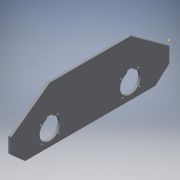
# Autodesk Inventor part: боковина
Saved by Autodesk Inventor 2019 (Build 230136000, 136)
## iProperties
Created: 2022-02-24
Part Number: боковина
Material: Типовые
Document SubType Name: Modeling
Designer: korsh
Density: 1 g/cm^3
Appearance: По умолчанию
Author: korsh
Autodesk Inventor part; units mm, degrees
ref_plane "YZ Plane" through (0, 0, 0) normal (1, 0, 0) x (0, 1, 0)
ref_plane "XZ Plane" through (0, 0, 0) normal (0, 1, 0) x (-1, 0, 0)
ref_plane "XY Plane" through (0, 0, 0) normal (0, 0, 1) x (1, 0, 0)
sketch "Эскиз1" plane through (0, 0, 0) normal (1, 0, 0) x (0, 1, 0)
  circle A0 centre (-34.2904, 95.1504) radius 32.5 projected
  circle A1 centre (-34.2904, 281.4981) radius 32.5 projected
  circle A2 centre (-13.0063, 263.3051) radius 2 projected
  circle A3 centre (-16.0973, 302.7822) radius 2 projected
  circle A4 centre (-55.5744, 299.6912) radius 2 projected
  circle A5 centre (-52.4834, 260.214) radius 2 projected
  circle A6 centre (-34.2904, 281.4981) radius 23.891 projected
  circle A7 centre (-34.2904, 95.1503) radius 23.891 projected
  circle A8 centre (-16.0973, 116.4344) radius 2 projected
  circle A9 centre (-13.0063, 76.9573) radius 2 projected
  circle A10 centre (-52.4834, 73.8663) radius 2 projected
  circle A11 centre (-55.5744, 113.3434) radius 2 projected
  arc A12 (-8.9692, 87.3685) -> (-6.9692, 89.3685) centre (-8.9692, 89.3685) ccw projected
  arc A13 (-6.9692, 100.7162) -> (-8.9692, 102.7162) centre (-8.9692, 100.7162) ccw projected
  line L0 (-6.9692, 89.3685) -> (-6.9692, 100.7162)
  line L1 (-8.9692, 87.3685) -> (-11.7023, 87.3685)
  line L2 (-8.9692, 102.7162) -> (-11.629, 102.7162)
  arc A14 (-58.1813, 281.4981) -> (-34.2904, 257.6071) centre (-34.2904, 281.4981) ccw projected
  arc A15 (-34.2904, 257.6071) -> (-14.7843, 267.7035) centre (-34.2904, 281.4981) ccw projected
  arc A16 (-14.7843, 267.7035) -> (-11.7023, 273.7162) centre (-34.2904, 281.4981) ccw projected
  line L3 (-11.7023, 273.7162) -> (-8.9692, 273.7162) projected
  arc A17 (-8.9692, 273.7162) -> (-6.9692, 275.7162) centre (-8.9692, 275.7162) ccw projected
  line L4 (-6.9692, 275.7162) -> (-6.9692, 280.4981) projected
  line L5 (-6.9692, 280.4981) -> (-6.9692, 282.4981) projected
  line L6 (-6.9692, 282.4981) -> (-6.9692, 287.064) projected
  arc A18 (-6.9692, 287.064) -> (-8.9692, 289.064) centre (-8.9692, 287.064) ccw projected
  line L7 (-8.9692, 289.064) -> (-11.629, 289.064) projected
  arc A19 (-11.629, 289.064) -> (-14.5225, 294.9149) centre (-34.2904, 281.4981) ccw projected
  arc A20 (-14.5225, 294.9149) -> (-34.2904, 305.3891) centre (-34.2904, 281.4981) ccw projected
  arc A21 (-34.2904, 305.3891) -> (-58.1813, 281.4981) centre (-34.2904, 281.4981) ccw projected
  circle A22 centre (-34.2904, 281.4981) radius 32.5 projected
  circle A23 centre (-52.4834, 260.214) radius 2 projected
  circle A24 centre (-13.0063, 263.3051) radius 2 projected
  circle A25 centre (-16.0973, 302.7822) radius 2 projected
  circle A26 centre (-55.5744, 299.6912) radius 2 projected
  line L8 (-6.9692, 100.7162) -> (-6.9692, 89.3685) projected
  line L9 (-8.9692, 87.3685) -> (-11.7023, 87.3685) projected
  line L10 (-11.629, 102.7162) -> (-8.9692, 102.7162) projected
  line L11 (-73.9692, 37.3685) -> (-73.9692, 339.064)
  circle A27 centre (-41.2904, 95.1504) radius 6 projected
  circle A28 centre (-41.2904, 281.4982) radius 6 projected
  line L12 (-41.2904, 5.1504) -> (-41.2904, 371.4982) construction
  line L13 (-73.9692, 37.3685) -> (-41.2904, 5.1504)
  line L14 (-73.9692, 339.064) -> (-41.2904, 371.4982)
  line L15 (-41.2904, 5.1504) -> (-6.2904, 5.1504)
  line L16 (-41.2904, 371.4982) -> (-6.2904, 371.4982)
  line L17 (-41.2904, 95.1504) -> (58.7096, 95.1504) construction
  line L18 (-41.2904, 281.4982) -> (58.7096, 281.4982) construction
  line L19 (-6.2904, 5.1504) -> (58.7096, 95.1504)
  line L20 (-6.2904, 371.4982) -> (58.7096, 281.4982)
  line L21 (58.7096, 95.1504) -> (58.7096, 281.4982)
  point P0 (0, 0)
  dimension "d0" = 67
  dimension "d1" = 50
  dimension "d2" = 67
  dimension "d3" = 50
  dimension "d4" = 90
  dimension "d6" = 90
  dimension "d7" = 34.3212
  dimension "d8" = 35
  dimension "d9" = 35
  dimension "d10" = 100
  constraints: 28 end point, 4 horizontal, 4 vertical, 2 point on circle, 1 parallel, 1 perpendicular
  measures "d0" distance between parallel lines of L11 L0
  measures "d1" distance from line of L11.start L1
  measures "d2" distance from line of L5.end L11
  measures "d3" distance from line of L7 L11.end
  measures "d4" distance of L12.start L17.start
  measures "d6" distance of L12.end L18.start
  measures "d7" distance from line of L17.start L0
  measures "d8" distance of L12.start L15.end
  measures "d9" distance of L12.end L16.end
  measures "d10" distance of L17.start L17.end
extrude "Выдавливание1" add sketch "Эскиз1" along normal blind 6 contours A0 | A1 | L11 L14 L16 L20 L21 L19 L15 L13
sketch "Эскиз2" plane through (0, 0, 0) normal (-1, 0, 0) x (0, 0, 1)
  point P0 (0, 0)
sketch "Эскиз3" plane through (6, 0, 0) normal (1, 0, 0) x (0, 0, -1)
  line L0 (-95.1504, 58.7096) -> (-281.4982, 58.7096) projected
  line L1 (-281.4982, 58.7096) -> (-271.4982, 58.7096)
  line L2 (-271.4982, 58.7096) -> (-271.4982, 52.7096)
  line L3 (-271.4982, 52.7096) -> (-281.4982, 52.7096)
  line L4 (-281.4982, 52.7096) -> (-281.4982, 58.7096)
  line L5 (-261.4982, 58.7096) -> (-251.4982, 58.7096)
  line L6 (-251.4982, 58.7096) -> (-251.4982, 52.7096)
  line L7 (-251.4982, 52.7096) -> (-261.4982, 52.7096)
  line L8 (-261.4982, 52.7096) -> (-261.4982, 58.7096)
  line L9 (-241.4982, 58.7096) -> (-231.4982, 58.7096)
  line L10 (-231.4982, 58.7096) -> (-231.4982, 52.7096)
  line L11 (-231.4982, 52.7096) -> (-241.4982, 52.7096)
  line L12 (-241.4982, 52.7096) -> (-241.4982, 58.7096)
  line L13 (-221.4982, 58.7096) -> (-211.4982, 58.7096)
  line L14 (-211.4982, 58.7096) -> (-211.4982, 52.7096)
  line L15 (-211.4982, 52.7096) -> (-221.4982, 52.7096)
  line L16 (-221.4982, 52.7096) -> (-221.4982, 58.7096)
  line L17 (-201.4982, 58.7096) -> (-191.4982, 58.7096)
  line L18 (-191.4982, 58.7096) -> (-191.4982, 52.7096)
  line L19 (-191.4982, 52.7096) -> (-201.4982, 52.7096)
  line L20 (-201.4982, 52.7096) -> (-201.4982, 58.7096)
  line L21 (-181.4982, 58.7096) -> (-171.4982, 58.7096)
  line L22 (-171.4982, 58.7096) -> (-171.4982, 52.7096)
  line L23 (-171.4982, 52.7096) -> (-181.4982, 52.7096)
  line L24 (-181.4982, 52.7096) -> (-181.4982, 58.7096)
  line L25 (-161.4982, 58.7096) -> (-151.4982, 58.7096)
  line L26 (-151.4982, 58.7096) -> (-151.4982, 52.7096)
  line L27 (-151.4982, 52.7096) -> (-161.4982, 52.7096)
  line L28 (-161.4982, 52.7096) -> (-161.4982, 58.7096)
  line L29 (-141.4982, 58.7096) -> (-131.4982, 58.7096)
  line L30 (-131.4982, 58.7096) -> (-131.4982, 52.7096)
  line L31 (-131.4982, 52.7096) -> (-141.4982, 52.7096)
  line L32 (-141.4982, 52.7096) -> (-141.4982, 58.7096)
  line L33 (-121.4982, 58.7096) -> (-111.4982, 58.7096)
  line L34 (-111.4982, 58.7096) -> (-111.4982, 52.7096)
  line L35 (-111.4982, 52.7096) -> (-121.4982, 52.7096)
  line L36 (-121.4982, 52.7096) -> (-121.4982, 58.7096)
  line L37 (-339.064, -73.9692) -> (-37.3685, -73.9692) projected
  line L38 (-333.064, -73.9692) -> (-323.064, -73.9692)
  line L39 (-323.064, -73.9692) -> (-323.064, -67.9692)
  line L40 (-323.064, -67.9692) -> (-333.064, -67.9692)
  line L41 (-333.064, -67.9692) -> (-333.064, -73.9692)
  line L42 (-359.8785, -5.2995) -> (-351.7717, 0.5554)
  line L43 (-351.7717, 0.5554) -> (-355.2846, 5.4194)
  line L44 (-355.2846, 5.4194) -> (-363.3914, -0.4355)
  line L45 (-363.3914, -0.4355) -> (-359.8785, -5.2995)
  line L46 (-359.8785, -5.2995) -> (-355.2846, 5.4194) construction
  line L47 (-351.7717, 0.5554) -> (-363.3914, -0.4355) construction
  line L48 (-281.4982, 58.7096) -> (-371.4982, -6.2904) projected
  line L49 (-335.5581, 12.2652) -> (-339.071, 17.1293)
  line L50 (-343.6649, 6.4103) -> (-335.5581, 12.2652)
  line L51 (-343.6649, 6.4103) -> (-339.071, 17.1293) construction
  line L52 (-339.071, 17.1293) -> (-347.1778, 11.2743)
  line L53 (-335.5581, 12.2652) -> (-347.1778, 11.2743) construction
  line L54 (-347.1778, 11.2743) -> (-343.6649, 6.4103)
  line L55 (-319.3445, 23.975) -> (-322.8574, 28.8391)
  line L56 (-327.4513, 18.1201) -> (-319.3445, 23.975)
  line L57 (-327.4513, 18.1201) -> (-322.8574, 28.8391) construction
  line L58 (-322.8574, 28.8391) -> (-330.9642, 22.9842)
  line L59 (-319.3445, 23.975) -> (-330.9642, 22.9842) construction
  line L60 (-330.9642, 22.9842) -> (-327.4513, 18.1201)
  line L61 (-303.1309, 35.6848) -> (-306.6438, 40.5489)
  line L62 (-311.2377, 29.8299) -> (-303.1309, 35.6848)
  line L63 (-311.2377, 29.8299) -> (-306.6438, 40.5489) construction
  line L64 (-306.6438, 40.5489) -> (-314.7506, 34.694)
  line L65 (-303.1309, 35.6848) -> (-314.7506, 34.694) construction
  line L66 (-314.7506, 34.694) -> (-311.2377, 29.8299)
  line L67 (-286.9173, 47.3946) -> (-290.4303, 52.2587)
  line L68 (-295.0241, 41.5397) -> (-286.9173, 47.3946)
  line L69 (-295.0241, 41.5397) -> (-290.4303, 52.2587) construction
  line L70 (-290.4303, 52.2587) -> (-298.5371, 46.4038)
  line L71 (-286.9173, 47.3946) -> (-298.5371, 46.4038) construction
  line L72 (-298.5371, 46.4038) -> (-295.0241, 41.5397)
  line L73 (-5.1504, -6.2904) -> (-95.1504, 58.7096) projected
  line L74 (-13.2572, -0.4355) -> (-16.7701, -5.2995)
  line L75 (-16.7701, -5.2995) -> (-24.8769, 0.5554)
  line L76 (-24.8769, 0.5554) -> (-21.364, 5.4194)
  line L77 (-21.364, 5.4194) -> (-13.2572, -0.4355)
  line L78 (-41.0905, 12.2652) -> (-37.5776, 17.1293)
  line L79 (-32.9837, 6.4103) -> (-41.0905, 12.2652)
  line L80 (-37.5776, 17.1293) -> (-29.4708, 11.2743)
  line L81 (-29.4708, 11.2743) -> (-32.9837, 6.4103)
  line L82 (-57.3041, 23.975) -> (-53.7912, 28.8391)
  line L83 (-49.1973, 18.1201) -> (-57.3041, 23.975)
  line L84 (-53.7912, 28.8391) -> (-45.6844, 22.9842)
  line L85 (-45.6844, 22.9842) -> (-49.1973, 18.1201)
  line L86 (-73.5177, 35.6848) -> (-70.0047, 40.5489)
  line L87 (-65.4109, 29.8299) -> (-73.5177, 35.6848)
  line L88 (-70.0047, 40.5489) -> (-61.898, 34.694)
  line L89 (-61.898, 34.694) -> (-65.4109, 29.8299)
  line L90 (-89.7313, 47.3946) -> (-86.2183, 52.2587)
  line L91 (-81.6245, 41.5397) -> (-89.7313, 47.3946)
  line L92 (-86.2183, 52.2587) -> (-78.1115, 46.4038)
  line L93 (-78.1115, 46.4038) -> (-81.6245, 41.5397)
  line L94 (-313.064, -73.9692) -> (-303.064, -73.9692)
  line L95 (-303.064, -73.9692) -> (-303.064, -67.9692)
  line L96 (-303.064, -67.9692) -> (-313.064, -67.9692)
  line L97 (-313.064, -67.9692) -> (-313.064, -73.9692)
  line L98 (-293.064, -73.9692) -> (-283.064, -73.9692)
  line L99 (-283.064, -73.9692) -> (-283.064, -67.9692)
  line L100 (-283.064, -67.9692) -> (-293.064, -67.9692)
  line L101 (-293.064, -67.9692) -> (-293.064, -73.9692)
  line L102 (-273.064, -73.9692) -> (-263.064, -73.9692)
  line L103 (-263.064, -73.9692) -> (-263.064, -67.9692)
  line L104 (-263.064, -67.9692) -> (-273.064, -67.9692)
  line L105 (-273.064, -67.9692) -> (-273.064, -73.9692)
  line L106 (-253.064, -73.9692) -> (-243.064, -73.9692)
  line L107 (-243.064, -73.9692) -> (-243.064, -67.9692)
  line L108 (-243.064, -67.9692) -> (-253.064, -67.9692)
  line L109 (-253.064, -67.9692) -> (-253.064, -73.9692)
  line L110 (-233.064, -73.9692) -> (-223.064, -73.9692)
  line L111 (-223.064, -73.9692) -> (-223.064, -67.9692)
  line L112 (-223.064, -67.9692) -> (-233.064, -67.9692)
  line L113 (-233.064, -67.9692) -> (-233.064, -73.9692)
  line L114 (-213.064, -73.9692) -> (-203.064, -73.9692)
  line L115 (-203.064, -73.9692) -> (-203.064, -67.9692)
  line L116 (-203.064, -67.9692) -> (-213.064, -67.9692)
  line L117 (-213.064, -67.9692) -> (-213.064, -73.9692)
  line L118 (-193.064, -73.9692) -> (-183.064, -73.9692)
  line L119 (-183.064, -73.9692) -> (-183.064, -67.9692)
  line L120 (-183.064, -67.9692) -> (-193.064, -67.9692)
  line L121 (-193.064, -67.9692) -> (-193.064, -73.9692)
  line L122 (-173.064, -73.9692) -> (-163.064, -73.9692)
  line L123 (-163.064, -73.9692) -> (-163.064, -67.9692)
  line L124 (-163.064, -67.9692) -> (-173.064, -67.9692)
  line L125 (-173.064, -67.9692) -> (-173.064, -73.9692)
  line L126 (-153.064, -73.9692) -> (-143.064, -73.9692)
  line L127 (-143.064, -73.9692) -> (-143.064, -67.9692)
  line L128 (-143.064, -67.9692) -> (-153.064, -67.9692)
  line L129 (-153.064, -67.9692) -> (-153.064, -73.9692)
  line L130 (-133.064, -73.9692) -> (-123.064, -73.9692)
  line L131 (-123.064, -73.9692) -> (-123.064, -67.9692)
  line L132 (-123.064, -67.9692) -> (-133.064, -67.9692)
  line L133 (-133.064, -67.9692) -> (-133.064, -73.9692)
  line L134 (-113.064, -73.9692) -> (-103.064, -73.9692)
  line L135 (-103.064, -73.9692) -> (-103.064, -67.9692)
  line L136 (-103.064, -67.9692) -> (-113.064, -67.9692)
  line L137 (-113.064, -67.9692) -> (-113.064, -73.9692)
  line L138 (-93.064, -73.9692) -> (-83.064, -73.9692)
  line L139 (-83.064, -73.9692) -> (-83.064, -67.9692)
  line L140 (-83.064, -67.9692) -> (-93.064, -67.9692)
  line L141 (-93.064, -67.9692) -> (-93.064, -73.9692)
  line L142 (-73.064, -73.9692) -> (-63.064, -73.9692)
  line L143 (-63.064, -73.9692) -> (-63.064, -67.9692)
  line L144 (-63.064, -67.9692) -> (-73.064, -67.9692)
  line L145 (-73.064, -67.9692) -> (-73.064, -73.9692)
  line L146 (-53.064, -73.9692) -> (-43.064, -73.9692)
  line L147 (-43.064, -73.9692) -> (-43.064, -67.9692)
  line L148 (-43.064, -67.9692) -> (-53.064, -67.9692)
  line L149 (-53.064, -67.9692) -> (-53.064, -73.9692)
  line L150 (-371.4982, -6.2904) -> (-365.4982, -6.2904)
  line L151 (-365.4982, -6.2904) -> (-365.4982, -16.2904)
  line L152 (-365.4982, -16.2904) -> (-371.4982, -16.2904)
  line L153 (-371.4982, -16.2904) -> (-371.4982, -6.2904)
  line L154 (-365.4982, -36.2904) -> (-371.4982, -36.2904)
  line L155 (-371.4982, -36.2904) -> (-371.4982, -26.2904)
  line L156 (-365.4982, -26.2904) -> (-365.4982, -36.2904)
  line L157 (-371.4982, -26.2904) -> (-365.4982, -26.2904)
  line L158 (-5.1504, -41.2904) -> (-5.1504, -6.2904) projected
  line L159 (-5.1504, -6.2904) -> (-11.1504, -6.2904)
  line L160 (-11.1504, -6.2904) -> (-11.1504, -16.2904)
  line L161 (-11.1504, -16.2904) -> (-5.1504, -16.2904)
  line L162 (-5.1504, -16.2904) -> (-5.1504, -6.2904)
  line L163 (-5.1504, -26.2904) -> (-11.1504, -26.2904)
  line L164 (-11.1504, -26.2904) -> (-11.1504, -36.2904)
  line L165 (-11.1504, -36.2904) -> (-5.1504, -36.2904)
  line L166 (-5.1504, -36.2904) -> (-5.1504, -26.2904)
  line L167 (-371.4982, -41.2904) -> (-339.064, -73.9692) projected
  line L168 (-37.3685, -73.9692) -> (-5.1504, -41.2904) projected
  line L169 (-365.4982, -47.3356) -> (-361.2396, -43.109)
  line L170 (-361.2396, -43.109) -> (-354.1952, -50.2066)
  line L171 (-354.1952, -50.2066) -> (-358.4537, -54.4332)
  line L172 (-365.4982, -47.3356) -> (-358.4537, -54.4332)
  line L173 (-347.1507, -57.3041) -> (-340.1063, -64.4017)
  line L174 (-351.4093, -61.5308) -> (-344.3648, -68.6284)
  line L175 (-340.1063, -64.4017) -> (-344.3648, -68.6284)
  line L176 (-351.4093, -61.5308) -> (-347.1507, -57.3041)
  line L177 (-11.0658, -47.2904) -> (-15.3385, -43.078)
  line L178 (-15.3385, -43.078) -> (-22.3592, -50.1991)
  line L179 (-22.3592, -50.1991) -> (-18.0865, -54.4115)
  line L180 (-11.0658, -47.2904) -> (-18.0865, -54.4115)
  line L181 (-25.1072, -61.5326) -> (-29.3798, -57.3201)
  line L182 (-29.3798, -57.3201) -> (-36.4005, -64.4412)
  line L183 (-36.4005, -64.4412) -> (-32.1279, -68.6537)
  line L184 (-25.1072, -61.5326) -> (-32.1279, -68.6537)
  point P0 (-357.5815, 0.0599)
  point P1 (-341.3679, 11.7698)
  point P2 (-325.1544, 23.4796)
  point P3 (-308.9408, 35.1894)
  point P4 (-292.7272, 46.8992)
  point P5 (-25.1918, -50.5326)
  dimension "d13" = 10
  dimension "d14" = 6
  dimension "d17" = 20
  dimension "d32" = 6
  dimension "d33" = 10
  dimension "d34" = 6
  dimension "d35" = 10
  dimension "d36" = 6
  dimension "d39" = 20
  dimension "d44" = 10
  dimension "d49" = 6
  dimension "d50" = 10
  dimension "d51" = 6
  dimension "d52" = 10
  dimension "d55" = 20
  dimension "d62" = 20
  dimension "d67" = 6
  dimension "d68" = 10
  dimension "d71" = 20
  dimension "d76" = 6
  dimension "d77" = 10
  dimension "d80" = 20
  dimension "d85" = 6
  dimension "d86" = 10
  dimension "d87" = 90
  dimension "d88" = 90
  dimension "d91" = 20
  dimension "d97" = 90
  dimension "d99" = 6
  dimension "d100" = 10
  dimension "d103" = 20
  dimension "d109" = 6
  dimension "d110" = 6
  constraints: 356 end point, 11 parallel, 10 midpoint, 8 perpendicular, 7 point on line, 6 horizontal, 4 collinear, 2 vertical, 288 other
  measures "d13" distance of L2.end L3.end
  measures "d14" distance of L1.end L2.end
  measures "d17" distance of L2.end L6.end
  measures "d32" distance of L38.end L39.end
  measures "d33" distance of L39.end L40.end
  measures "d34" distance from line of L37.start L41
  measures "d35" distance of L43.end L44.end
  measures "d36" distance of L44.end L42.start
  measures "d39" distance of L42.end L49.start
  measures "d44" distance from line of L45 L48.end
  measures "d49" distance of L74.start L74.end
  measures "d50" distance of L74.end L75.end
  measures "d51" distance of L75.end L76.end
  measures "d52" distance from line of L73.start L74
  measures "d55" distance of L75.end L78.start
  measures "d62" distance of L38.start L94.start
  measures "d67" distance of L151.end L152.end
  measures "d68" distance of L150.end L151.end
  measures "d71" distance of L152.end L154.end
  measures "d76" distance of L161.end L160.end
  measures "d77" distance of L160.end L159.end
  measures "d80" distance of L159.end L163.end
  measures "d85" distance of L169.start L169.end
  measures "d86" distance of L169.end L170.end
  measures "d87" angle of L167 L169
  measures "d88" angle of L170 L169
  measures "d91" distance of L169.end L173.start
  measures "d97" angle of L168 L177
  measures "d99" distance of L177.start L177.end
  measures "d100" distance of L177.end L178.end
  measures "d103" distance of L164.end point (-25.192, -50.533)
  measures "d109" horizontal distance of L169.start L167.start
  measures "d110" vertical distance of L158.start L177.start
extrude "Выдавливание2" cut sketch "Эскиз3" against normal blind 6
equation "\"d6\" = d4"
equation "\"d52\" = d44"
